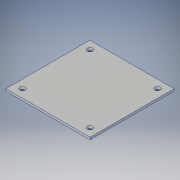
# Autodesk Inventor part: Piston Build surface
Saved by Autodesk Inventor 2018 (Build 220112000, 112)
## iProperties
Created: 2013-10-18
Part Number: Piston Build surface
Material: Aluminum 6061
Document SubType Name: Modeling
Designer: Gabriel Smolnycki
Mass: 240.071 g
Surface Area: 471.415 cm^2
Volume: 88.9152 cm^3
Density: 2.7 g/cm^3
Appearance: Aluminum - Flat
Sending System: SolidWorks 2017
Last Author: Gabriel Smolnycki
Last Saved: 2017-09-14
Author: Gabriel Smolnycki
Autodesk Inventor part; units mm, degrees
ref_plane "YZ Plane" through (0, 0, 0) normal (1, 0, 0) x (0, 1, 0)
ref_plane "XZ Plane" through (0, 0, 0) normal (0, 1, 0) x (-1, 0, 0)
ref_plane "XY Plane" through (0, 0, 0) normal (0, 0, 1) x (1, 0, 0)
sketch "Sketch1" plane through (0, 0, 0) normal (0, 1, 0) x (-1, 0, 0)
  line L0 (74.75, 74.575) -> (-74.75, 74.575)
  line L1 (-74.75, 74.575) -> (-74.75, -74.575)
  line L2 (-74.75, -74.575) -> (74.75, -74.575)
  line L3 (74.75, -74.575) -> (74.75, 74.575)
  line L4 (74.75, 74.575) -> (-74.75, -74.575) construction
  line L5 (-74.75, 74.575) -> (74.75, -74.575) construction
  point P0 (0, 0)
  dimension "d32" = 149.5
  dimension "d33" = 149.15
  constraints: 12 end point, 2 midpoint, 2 parallel, 1 horizontal, 1 perpendicular
  measures "d32" distance of L2.end L1.end
  measures "d33" distance of L1.end L0.end
extrude "Extrusion1" add sketch "Sketch1" against normal blind 4.064
hole "Hole4" at (60, 0, -60) direction (0, -1, 0) diameter 4.5 depth 4.064 countersink diameter 9.4 countersink angle 90
hole "Hole3" at (-60, 0, 60) direction (0, -1, 0) diameter 4.5 depth 4.064 countersink diameter 9.4 countersink angle 90
sketch "Sketch3" plane through (0, 0, 0) normal (0, 1, 0) x (-1, 0, 0)
  point P0 (60, 60)
hole "Hole2" at (60, 0, 60) direction (0, -1, 0) diameter 4.5 depth 4.064 countersink diameter 9.4 countersink angle 90
sketch "Sketch2" plane through (0, 0, 0) normal (0, 1, 0) x (-1, 0, 0)
  point P0 (-60, -60)
hole "Hole1" at (-60, 0, -60) direction (0, -1, 0) diameter 4.5 depth 4.064 countersink diameter 9.4 countersink angle 90
sketch "Sketch4" plane through (0, 0, 0) normal (0, 1, 0) x (-1, 0, 0)
  point P0 (-60, 60)
sketch "Sketch5" plane through (0, 0, 0) normal (0, 1, 0) x (-1, 0, 0)
  point P0 (60, -60)
body "Solid3"
